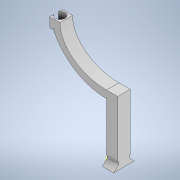
# Autodesk Inventor part: Pasteur_holderNEW
Saved by Autodesk Inventor 2020 (Build 240168000, 168)
## iProperties
Created: 2020-11-04
Part Number: Pasteur_holderNEW
Material: Generic
Document SubType Name: Modeling
Designer: Allesfresser
Density: 1 g/cm^3
Appearance: Default
Author: Allesfresser
Autodesk Inventor part; units mm, degrees
ref_plane "YZ Plane" through (0, 0, 0) normal (1, 0, 0) x (0, 1, 0)
ref_plane "XZ Plane" through (0, 0, 0) normal (0, 1, 0) x (-1, 0, 0)
ref_plane "XY Plane" through (0, 0, 0) normal (0, 0, 1) x (1, 0, 0)
sketch "Sketch1" plane through (0, 0, 0) normal (1, 0, 0) x (0, 1, 0)
  line L0 (0, 0) -> (0, 3.9)
  line L1 (0, 0) -> (0, -3.9)
  line L2 (0, 3.9) -> (-3.3941, 7.2941)
  line L3 (0, 3.9) -> (4.8, 3.9) construction
  line L4 (0, -3.9) -> (-3.3941, -7.2941)
  line L5 (0, -3.9) -> (4.8, -3.9) construction
  line L6 (-3.3941, -7.2941) -> (-3.3941, 7.2941)
  dimension "d0" = 3.9
  dimension "d1" = 3.9
  dimension "d2" = 4.8
  dimension "d3" = 135
  dimension "d4" = 4.8
  dimension "d5" = 135
  constraints: 14 end point, 2 equal length, 2 horizontal, 2 vertical
  measures "d0" distance of L0.start L0.end
  measures "d1" distance of L0.start L1.end
  measures "d2" distance of L0.end L2.end
  measures "d3" angle of L3 L2
  measures "d4" distance of L1.end L4.end
  measures "d5" angle of L4 L5
extrude "Extrusion1" add sketch "Sketch1" along normal blind 8
sketch "Sketch2" plane through (0, 0, 3.9) normal (0, 1, 0) x (1, 0, 0)
  line L0 (0, -3.3941) -> (0, 11.1941) projected
  line L1 (0, -0.0082) -> (8, -0.0082)
  line L2 (8, -0.0082) -> (8, 7.7918)
  line L3 (8, 7.7918) -> (0, 7.7918)
  line L4 (0, 7.7918) -> (0, -0.0082)
  point P0 (0, 3.9)
  dimension "d8" = 8
  dimension "d9" = 7.8
  constraints: 8 end point, 2 parallel, 1 horizontal, 1 perpendicular, 1 point on line
  measures "d8" distance of L3.end L2.end
  measures "d9" distance of L2.end L1.end
extrude "Extrusion2" add sketch "Sketch2" along normal blind 2
sketch "Sketch3" plane through (0, 2, 3.9) normal (0, 1, 0) x (1, 0, 0)
  line L0 (8, -0.5082) -> (0, -0.5082)
  line L1 (0, -0.5082) -> (0, 8.2918)
  line L2 (0, 8.2918) -> (8, 8.2918)
  line L3 (8, 8.2918) -> (8, -0.5082)
  line L4 (8, -0.5082) -> (0, 8.2918) construction
  line L5 (0, -0.5082) -> (8, 8.2918) construction
  line L6 (8, 7.7918) -> (0, 7.7918) projected
  point P0 (0, 3.9)
  point P1 (4, 3.8918)
  dimension "d12" = 8
  dimension "d13" = 8.8
  dimension "d14" = 3.9
  dimension "d15" = 4
  constraints: 12 end point, 2 midpoint, 2 parallel, 1 horizontal, 1 perpendicular
  measures "d12" distance of L1.end L2.end
  measures "d13" distance of L0.end L1.end
  measures "d14" distance from line of L6 point (4, 3.892)
  measures "d15" distance of point (0, 3.9) point (4, 3.892)
extrude "Extrusion3" add sketch "Sketch3" along normal blind 64.606
sketch "Sketch4" plane through (0, 0, 0) normal (-1, 0, 0) x (0, 0, 1)
  line L0 (-4.3918, 2) -> (-4.3918, 66.606) projected
  line L1 (4.4082, 2) -> (4.4082, 66.606) projected
  line L2 (-4.3918, 66.606) -> (4.4082, 66.606)
  line L3 (4.4082, 66.606) -> (4.4082, 36.606)
  line L4 (4.4082, 36.606) -> (-4.3918, 36.606)
  line L5 (-4.3918, 36.606) -> (-4.3918, 66.606)
  point P0 (0, 0)
  point P1 (-4.3918, 36.606)
  dimension "d18" = 30
  constraints: 8 end point, 2 parallel, 1 horizontal, 1 perpendicular, 1 point on line
  measures "d18" distance of L2.end L3.end
extrude "Extrusion4" add sketch "Sketch4" along normal blind 40
sketch "Sketch5" plane through (0, 66.606, 3.9) normal (0, 1, 0) x (1, 0, 0)
  circle A0 centre (-37, 3.8918) radius 3.45
  line L0 (-40, -0.5082) -> (-40, 8.2918) projected
  point P0 (0, 3.9)
  point P1 (-40, 5.5955)
  point P2 (-40, 2.1882)
  dimension "d21" = 6.9
  dimension "d22" = 3
  constraints: 1 centre point
  measures "d21" diameter of A0
  measures "d22" distance from line of A0.centre L0
sketch "Sketch6" plane through (0, 2, 4.4082) normal (0, 0, 1) x (1, 0, 0)
  point P0 (0, -2)
sketch "Sketch7" plane through (0, 2, 4.4082) normal (0, 0, 1) x (1, 0, 0)
  point P0 (0, -2)
sketch "Sketch10" plane through (0, 2, 4.4082) normal (0, 0, 1) x (1, 0, 0)
  ellipse E0 centre (0, 64.6805) end of major axis (0, 39.8349) minor radius 32.7521
  line L0 (8, 64.606) -> (-40, 64.606) projected
  line L1 (0, 39.8349) -> (8, 39.8349)
  line L2 (8, 39.8349) -> (8, 64.606)
  line L3 (8, 64.606) -> (0, 64.606)
  line L4 (0, 64.606) -> (0, 39.8349)
  point P0 (0, -2)
  point P1 (8, 40.5875)
  constraints: 8 end point, 2 parallel, 1 horizontal, 1 perpendicular, 3 other
extrude "Extrusion8" cut sketch "Sketch10" against normal blind 10
sketch "Sketch13" plane through (0, 36.606, -4.3918) normal (0, -1, 0) x (1, 0, 0)
  circle A0 centre (-37.1694, 4.3918) radius 4.375
  point P0 (0, 4.3918)
  dimension "d37" = 8.75
  constraints: 1 centre point
  measures "d37" diameter of A0
extrude "Extrusion9" cut sketch "Sketch13" against normal blind 24
extrude "Extrusion10" cut sketch "Sketch5" against normal blind 24
sketch "Sketch14" plane through (8, 2, -4.3918) normal (0, 0, -1) x (-1, 0, 0)
  line L0 (48, 34.606) -> (40.7944, 34.606) projected
  line L1 (45.2609, 34.606) -> (48, 34.606)
  line L2 (48, 34.606) -> (48, 57.8825)
  line L3 (48, 57.8825) -> (45.2609, 57.8825)
  line L4 (45.2609, 57.8825) -> (45.2609, 34.606)
  point P0 (8, -2)
  constraints: 8 end point, 2 parallel, 1 horizontal, 1 perpendicular, 1 point on line
extrude "Extrusion11" cut sketch "Sketch14" against normal blind 24
sketch "Sketch15" plane through (0, 2, 4.4082) normal (0, 0, 1) x (1, 0, 0)
  line L0 (-37.2609, 57.8825) -> (-37.2609, 34.606) projected
  line L1 (0, 34.606) -> (-37.2609, 34.606) projected
  arc A0 (-37.2609, 57.8825) -> (0, 34.606) centre (-0.1523, 75.824) ccw
  point P0 (0, -2)
  point P1 (-0.3046, 34.606)
  constraints: 2 point on circle, 1 centre point
extrude "Extrusion12" cut sketch "Sketch15" against normal through all
body "Solid1"
